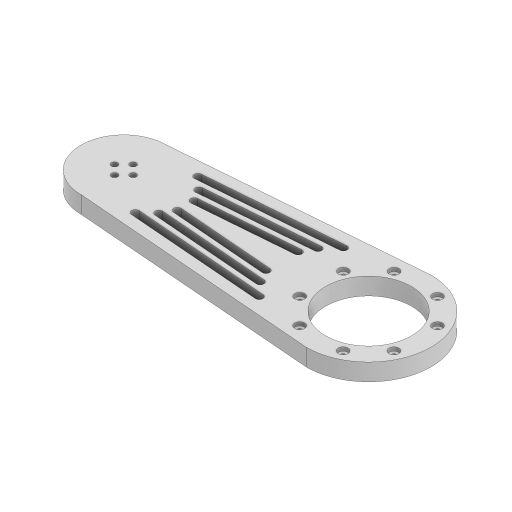
# Autodesk Inventor part: Link1
Saved by Autodesk Inventor 2024.3 (Build 283343000, 343)
## iProperties
Created: 2025-09-03
Part Number: Link1
Material: Generic
Document SubType Name: Modeling
Designer: danie
Density: 1 g/cm^3
Appearance: Default
Author: danie
Autodesk Inventor part; units mm, degrees
ref_plane "YZ Plane" through (0, 0, 0) normal (1, 0, 0) x (0, 1, 0)
ref_plane "XZ Plane" through (0, 0, 0) normal (0, 1, 0) x (-1, 0, 0)
ref_plane "XY Plane" through (0, 0, 0) normal (0, 0, 1) x (1, 0, 0)
sketch "Block1" plane through (0, 0, 0) normal (0, 0, 1) x (1, 0, 0)
  circle A0 centre (7.5478, 0.0598) radius 3.1
  circle A1 centre (-7.6522, 0.0598) radius 3.1
  circle A2 centre (-0.0522, 0.0598) radius 15.1
  circle A3 centre (-0.0522, 7.6598) radius 3.1
  circle A4 centre (-0.0522, -7.5402) radius 3.1
  point P0 (-0.0522, 0.0598)
sketch "Block2" plane through (0, 0, 0) normal (0, 0, 1) x (1, 0, 0)
  arc A0 (-125.615, -182.0442) -> (-128.3642, -184.6132) centre (-121.6807, -189.0099) ccw
  circle A1 centre (-125.7842, -178.7986) radius 1.5875
  circle A2 centre (-125.7842, -178.7986) radius 1.5875
  arc A3 (-123.2766, -176.7312) -> (-125.615, -182.0442) centre (-125.7842, -178.7986) ccw
  circle A4 centre (-125.7842, -178.7986) radius 3.25
  arc A5 (-140.9961, -137.689) -> (-141.0844, -134.7775) centre (-142.4103, -136.2748) ccw
  arc A6 (-128.2959, -137.4522) -> (-140.6552, -125.0571) centre (-164.2878, -160.9806) ccw
  arc A7 (-141.0844, -134.7775) -> (-153.1968, -127.7844) centre (-164.2878, -160.9806) ccw
  arc A8 (-143.2242, -122.3079) -> (-140.6552, -125.0571) centre (-136.2585, -118.3736) ccw
  circle A9 centre (-146.4698, -122.4771) radius 1.5875
  circle A10 centre (-146.4698, -122.4771) radius 1.5875
  arc A11 (-148.4415, -119.8935) -> (-143.2242, -122.3079) centre (-146.4698, -122.4771) ccw
  circle A12 centre (-146.4698, -122.4771) radius 3.25
  arc A13 (-152.1999, -119.7146) -> (-148.4415, -119.8935) centre (-149.951, -112.0372) ccw
  arc A14 (-202.9605, -139.9171) -> (-200.2113, -137.3481) centre (-206.8948, -132.9514) ccw
  circle A15 centre (-202.7913, -143.1627) radius 1.5875
  circle A16 centre (-202.7913, -143.1627) radius 1.5875
  arc A17 (-205.3749, -145.1344) -> (-202.9605, -139.9171) centre (-202.7913, -143.1627) ccw
  circle A18 centre (-202.7913, -143.1627) radius 3.25
  arc A19 (-150.7156, -144.8249) -> (-148.0149, -144.7078) centre (-149.4291, -143.2936) ccw
  line L0 (-140.9961, -137.689) -> (-148.0149, -144.7078)
  line L1 (-142.0587, -155.0244) -> (-132.4708, -152.4553)
  arc A20 (-142.0587, -155.0244) -> (-143.5104, -157.3047) centre (-141.541, -156.9562) ccw
  arc A21 (-177.8599, -177.1363) -> (-180.5606, -177.2535) centre (-179.1464, -178.6677) ccw
  arc A22 (-176.3756, -202.2467) -> (-180.134, -202.0677) centre (-178.6245, -209.924) ccw
  arc A23 (-175.3787, -194.1769) -> (-172.8131, -192.7976) centre (-174.7449, -192.28) ccw
  arc A24 (-177.8599, -177.1363) -> (-171.4929, -180.8123) centre (-164.2878, -160.9806) ccw
  line L2 (-170.244, -183.2097) -> (-172.8131, -192.7976)
  arc A25 (-170.244, -183.2097) -> (-171.4929, -180.8123) centre (-172.1759, -182.6921) ccw
  arc A26 (-157.0826, -180.8123) -> (-158.3315, -183.2097) centre (-156.3996, -182.6921) ccw
  line L3 (-155.7624, -192.7976) -> (-158.3315, -183.2097)
  arc A27 (-157.0826, -180.8123) -> (-150.7156, -177.1363) centre (-164.2878, -160.9806) ccw
  arc A28 (-155.7624, -192.7976) -> (-153.1968, -194.1769) centre (-153.8306, -192.28) ccw
  arc A29 (-176.3756, -202.2467) -> (-152.3193, -202.2815) centre (-164.2878, -160.9806) ccw
  arc A30 (-200.2796, -184.5091) -> (-203.4208, -181.7197) centre (-206.9757, -188.8865) ccw
  circle A31 centre (-202.8427, -178.6871) radius 1.5875
  arc A32 (-205.5197, -177.1495) -> (-205.5886, -172.9491) centre (-213.2724, -175.1758) ccw
  arc A33 (-205.5197, -177.1495) -> (-203.4208, -181.7197) centre (-201.6434, -178.1363) ccw
  arc A34 (-187.712, -124.9209) -> (-200.2113, -137.3481) centre (-164.2878, -160.9806) ccw
  arc A35 (-187.4911, -134.7775) -> (-187.5794, -137.689) centre (-186.1652, -136.2748) ccw
  line L4 (-180.5606, -144.7078) -> (-187.5794, -137.689)
  arc A36 (-180.5606, -144.7078) -> (-177.8599, -144.8249) centre (-179.1464, -143.2936) ccw
  arc A37 (-171.4929, -141.149) -> (-177.8599, -144.8249) centre (-164.2878, -160.9806) ccw
  arc A38 (-175.3787, -127.7844) -> (-187.4911, -134.7775) centre (-164.2878, -160.9806) ccw
  arc A39 (-171.4929, -141.149) -> (-170.244, -138.7515) centre (-172.1759, -139.2692) ccw
  arc A40 (-172.8131, -129.1637) -> (-175.3787, -127.7844) centre (-174.7449, -129.6813) ccw
  line L5 (-172.8131, -129.1637) -> (-170.244, -138.7515)
  arc A41 (-140.8512, -197.0324) -> (-128.3642, -184.6132) centre (-164.2878, -160.9806) ccw
  arc A42 (-141.0844, -187.1838) -> (-140.9961, -184.2723) centre (-142.4103, -185.6865) ccw
  line L6 (-148.0149, -177.2535) -> (-140.9961, -184.2723)
  arc A43 (-148.0149, -177.2535) -> (-150.7156, -177.1363) centre (-149.4291, -178.6677) ccw
  arc A44 (-140.8512, -197.0324) -> (-143.6285, -200.1265) centre (-136.4909, -203.7397) ccw
  arc A45 (-153.1968, -194.1769) -> (-141.0844, -187.1838) centre (-164.2878, -160.9806) ccw
  circle A46 centre (-146.5813, -199.5355) radius 1.5875
  arc A47 (-148.1624, -202.2017) -> (-143.6285, -200.1265) centre (-147.1972, -198.3199) ccw
  arc A48 (-148.1624, -202.2017) -> (-152.3193, -202.2815) centre (-150.0927, -209.9653) ccw
  arc A49 (-150.7156, -144.8249) -> (-157.0826, -141.149) centre (-164.2878, -160.9806) ccw
  arc A50 (-158.3315, -138.7515) -> (-157.0826, -141.149) centre (-156.3996, -139.2692) ccw
  line L7 (-158.3315, -138.7515) -> (-155.7624, -129.1637)
  arc A51 (-153.1968, -127.7844) -> (-155.7624, -129.1637) centre (-153.8306, -129.6813) ccw
  arc A52 (-187.712, -124.9209) -> (-184.9593, -121.878) centre (-192.07, -118.2121) ccw
  circle A53 centre (-181.9942, -122.4257) radius 1.5875
  arc A54 (-180.4775, -119.8197) -> (-184.9593, -121.878) centre (-181.404, -123.7109) ccw
  arc A55 (-180.4775, -119.8197) -> (-176.3756, -119.7146) centre (-178.6245, -112.0372) ccw
  arc A56 (-152.1999, -119.7146) -> (-176.3756, -119.7146) centre (-164.2878, -160.9806) ccw
  arc A57 (-128.2959, -137.4522) -> (-125.1547, -140.2416) centre (-121.5998, -133.0748) ccw
  circle A58 centre (-125.7329, -143.2742) radius 1.5875
  arc A59 (-123.0558, -144.8118) -> (-125.1547, -140.2416) centre (-126.9321, -143.8249) ccw
  arc A60 (-123.0558, -144.8118) -> (-122.9869, -149.0122) centre (-115.3031, -146.7855) ccw
  line L8 (-132.4708, -169.506) -> (-142.0587, -166.9369)
  arc A61 (-143.5104, -164.6566) -> (-142.0587, -166.9369) centre (-141.541, -165.0051) ccw
  arc A62 (-143.5104, -164.6566) -> (-143.5104, -157.3047) centre (-164.2878, -160.9806) ccw
  arc A63 (-129.9935, -153.9876) -> (-132.4708, -152.4553) centre (-131.9532, -154.3872) ccw
  arc A64 (-129.9935, -167.9737) -> (-129.9935, -153.9876) centre (-164.2878, -160.9806) ccw
  arc A65 (-132.4708, -169.506) -> (-129.9935, -167.9737) centre (-131.9532, -167.5741) ccw
  arc A66 (-123.0527, -173.1738) -> (-122.9869, -149.0122) centre (-164.2878, -160.9806) ccw
  arc A67 (-123.0527, -173.1738) -> (-123.2766, -176.7312) centre (-115.3811, -175.4423) ccw
  arc A68 (-205.5538, -148.8928) -> (-205.3749, -145.1344) centre (-213.2312, -146.6439) ccw
  arc A69 (-196.1047, -152.4553) -> (-198.582, -153.9876) centre (-196.6224, -154.3872) ccw
  line L9 (-196.1047, -152.4553) -> (-186.5169, -155.0244)
  arc A70 (-185.0651, -157.3047) -> (-186.5169, -155.0244) centre (-187.0345, -156.9562) ccw
  circle A71 centre (-164.2878, -160.9806) radius 15.5
  arc A72 (-185.0651, -157.3047) -> (-185.0651, -164.6566) centre (-164.2878, -160.9806) ccw
  arc A73 (-186.5169, -166.9369) -> (-185.0651, -164.6566) centre (-187.0345, -165.0051) ccw
  line L10 (-186.5169, -166.9369) -> (-196.1047, -169.506)
  arc A74 (-198.582, -153.9876) -> (-198.582, -167.9737) centre (-164.2878, -160.9806) ccw
  arc A75 (-205.5538, -148.8928) -> (-205.5886, -172.9491) centre (-164.2878, -160.9806) ccw
  arc A76 (-198.582, -167.9737) -> (-196.1047, -169.506) centre (-196.6224, -167.5741) ccw
  circle A77 centre (-182.1057, -199.4842) radius 1.5875
  circle A78 centre (-182.1057, -199.4842) radius 1.5875
  arc A79 (-187.4911, -187.1838) -> (-175.3787, -194.1769) centre (-164.2878, -160.9806) ccw
  arc A80 (-180.134, -202.0677) -> (-185.3513, -199.6534) centre (-182.1057, -199.4842) ccw
  circle A81 centre (-182.1057, -199.4842) radius 3.25
  arc A82 (-185.3513, -199.6534) -> (-187.9203, -196.9042) centre (-192.317, -203.5877) ccw
  arc A83 (-187.5794, -184.2723) -> (-187.4911, -187.1838) centre (-186.1652, -185.6865) ccw
  arc A84 (-200.2796, -184.5091) -> (-187.9203, -196.9042) centre (-164.2878, -160.9806) ccw
  line L11 (-187.5794, -184.2723) -> (-180.5606, -177.2535)
  point P0 (-164.2909, -160.9825)
sketch "Sketch1" plane through (0, 0, 0) normal (0, 1, 0) x (-1, 0, 0)
  circle A0 centre (0, 0) radius 15.1
  circle A1 centre (0, 0) radius 35
  line L0 (0, 0) -> (-200, 0)
  circle A2 centre (-200, 0) radius 15.5
  circle A3 centre (-200, 0) radius 51
  line L1 (0, 0) -> (0, 35)
  line L2 (0, 0) -> (0, -35)
  line L3 (-200, 0) -> (-200, 51)
  line L4 (-200, 0) -> (-200, -51)
  line L5 (0, 35) -> (-200, 51)
  line L6 (0, -35) -> (-200, -51)
  line L7 (-35, 25.6) -> (-145, 34.4) construction
  line L8 (-35.2392, 22.6096) -> (-145.2392, 31.4096)
  line L9 (-144.7608, 37.3904) -> (-34.7608, 28.5904)
  arc A4 (-35.2392, 22.6096) -> (-34.7608, 28.5904) centre (-35, 25.6) ccw
  arc A5 (-144.7608, 37.3904) -> (-145.2392, 31.4096) centre (-145, 34.4) ccw
  line L10 (-45, 16.4) -> (-135, 23.6) construction
  line L11 (-44.7608, 19.3904) -> (-134.7608, 26.5904)
  line L12 (-135.2392, 20.6096) -> (-45.2392, 13.4096)
  arc A6 (-45.2392, 13.4096) -> (-44.7608, 19.3904) centre (-45, 16.4) ccw
  arc A7 (-134.7608, 26.5904) -> (-135.2392, 20.6096) centre (-135, 23.6) ccw
  line L13 (-50.6641, 6.8531) -> (-129.3359, 13.1469) construction
  line L14 (-50.4249, 9.8436) -> (-129.0966, 16.1373)
  line L15 (-129.5751, 10.1564) -> (-50.9034, 3.8627)
  arc A8 (-50.9034, 3.8627) -> (-50.4249, 9.8436) centre (-50.6641, 6.8531) ccw
  arc A9 (-129.0966, 16.1373) -> (-129.5751, 10.1564) centre (-129.3359, 13.1469) ccw
  line L16 (-35.2392, -22.6096) -> (-145.2392, -31.4096)
  line L17 (-144.7608, -37.3904) -> (-34.7608, -28.5904)
  arc A10 (-34.7608, -28.5904) -> (-35.2392, -22.6096) centre (-35, -25.6) ccw
  arc A11 (-145.2392, -31.4096) -> (-144.7608, -37.3904) centre (-145, -34.4) ccw
  line L18 (-44.7608, -19.3904) -> (-134.7608, -26.5904)
  line L19 (-135.2392, -20.6096) -> (-45.2392, -13.4096)
  arc A12 (-44.7608, -19.3904) -> (-45.2392, -13.4096) centre (-45, -16.4) ccw
  arc A13 (-135.2392, -20.6096) -> (-134.7608, -26.5904) centre (-135, -23.6) ccw
  line L20 (-50.4249, -9.8436) -> (-129.0966, -16.1373)
  line L21 (-129.5751, -10.1564) -> (-50.9034, -3.8627)
  arc A14 (-50.4249, -9.8436) -> (-50.9034, -3.8627) centre (-50.6641, -6.8531) ccw
  arc A15 (-129.5751, -10.1564) -> (-129.0966, -16.1373) centre (-129.3359, -13.1469) ccw
  circle A16 centre (-200, 0) radius 35
  circle A17 centre (7.6, 0) radius 1.5
  circle A18 centre (0, 7.6) radius 1.5
  circle A19 centre (-7.6, 0) radius 1.5
  circle A20 centre (0, -7.6) radius 1.5
  circle A21 centre (7.6, 0) radius 3.1
  circle A22 centre (-7.6, 0) radius 3.1
  circle A23 centre (0, 0) radius 15.1
  circle A24 centre (0, 7.6) radius 3.1
  circle A25 centre (0, -7.6) radius 3.1
  arc A26 (-161.3273, -21.0635) -> (-164.0764, -23.6325) centre (-157.393, -28.0293) ccw
  circle A27 centre (-161.4965, -17.8179) radius 1.5875
  circle A28 centre (-161.4965, -17.8179) radius 1.5875
  arc A29 (-158.9888, -15.7505) -> (-161.3273, -21.0635) centre (-161.4965, -17.8179) ccw
  circle A30 centre (-161.4965, -17.8179) radius 3.25
  arc A31 (-176.7084, 23.2916) -> (-176.7967, 26.2032) centre (-178.1226, 24.7058) ccw
  arc A32 (-164.0082, 23.5285) -> (-176.3675, 35.9236) centre (-200, 0) ccw
  arc A33 (-176.7967, 26.2032) -> (-188.9091, 33.1962) centre (-200, 0) ccw
  arc A34 (-178.9365, 38.6727) -> (-176.3675, 35.9236) centre (-171.9707, 42.607) ccw
  circle A35 centre (-182.1821, 38.5035) radius 1.5875
  circle A36 centre (-182.1821, 38.5035) radius 1.5875
  arc A37 (-184.1537, 41.0871) -> (-178.9365, 38.6727) centre (-182.1821, 38.5035) ccw
  circle A38 centre (-182.1821, 38.5035) radius 3.25
  arc A39 (-187.9121, 41.266) -> (-184.1537, 41.0871) centre (-185.6632, 48.9434) ccw
  arc A40 (-238.6727, 21.0635) -> (-235.9236, 23.6325) centre (-242.607, 28.0293) ccw
  circle A41 centre (-238.5035, 17.8179) radius 1.5875
  circle A42 centre (-238.5035, 17.8179) radius 1.5875
  arc A43 (-241.0871, 15.8463) -> (-238.6727, 21.0635) centre (-238.5035, 17.8179) ccw
  circle A44 centre (-238.5035, 17.8179) radius 3.25
  arc A45 (-186.4278, 16.1557) -> (-183.7272, 16.2728) centre (-185.1414, 17.687) ccw
  line L22 (-176.7084, 23.2916) -> (-183.7272, 16.2728)
  line L23 (-177.7709, 5.9563) -> (-168.183, 8.5253)
  arc A46 (-177.7709, 5.9563) -> (-179.2227, 3.676) centre (-177.2533, 4.0244) ccw
  arc A47 (-213.5722, -16.1557) -> (-216.2728, -16.2728) centre (-214.8586, -17.687) ccw
  arc A48 (-212.0879, -41.266) -> (-215.8463, -41.0871) centre (-214.3368, -48.9434) ccw
  arc A49 (-211.0909, -33.1962) -> (-208.5253, -31.817) centre (-210.4572, -31.2993) ccw
  arc A50 (-213.5722, -16.1557) -> (-207.2052, -19.8317) centre (-200, 0) ccw
  line L24 (-205.9563, -22.2291) -> (-208.5253, -31.817)
  arc A51 (-205.9563, -22.2291) -> (-207.2052, -19.8317) centre (-207.8881, -21.7115) ccw
  arc A52 (-192.7948, -19.8317) -> (-194.0437, -22.2291) centre (-192.1119, -21.7115) ccw
  line L25 (-191.4747, -31.817) -> (-194.0437, -22.2291)
  arc A53 (-192.7948, -19.8317) -> (-186.4278, -16.1557) centre (-200, 0) ccw
  arc A54 (-191.4747, -31.817) -> (-188.9091, -33.1962) centre (-189.5428, -31.2993) ccw
  arc A55 (-212.0879, -41.266) -> (-188.0316, -41.3008) centre (-200, 0) ccw
  arc A56 (-235.9918, -23.5285) -> (-239.1331, -20.7391) centre (-242.688, -27.9059) ccw
  circle A57 centre (-238.5549, -17.7065) radius 1.5875
  arc A58 (-241.232, -16.1688) -> (-241.3008, -11.9684) centre (-248.9847, -14.1951) ccw
  arc A59 (-241.232, -16.1688) -> (-239.1331, -20.7391) centre (-237.3556, -17.1557) ccw
  arc A60 (-223.4243, 36.0597) -> (-235.9236, 23.6325) centre (-200, 0) ccw
  arc A61 (-223.2033, 26.2032) -> (-223.2916, 23.2916) centre (-221.8774, 24.7058) ccw
  line L26 (-216.2728, 16.2728) -> (-223.2916, 23.2916)
  arc A62 (-216.2728, 16.2728) -> (-213.5722, 16.1557) centre (-214.8586, 17.687) ccw
  arc A63 (-207.2052, 19.8317) -> (-213.5722, 16.1557) centre (-200, 0) ccw
  arc A64 (-211.0909, 33.1962) -> (-223.2033, 26.2032) centre (-200, 0) ccw
  arc A65 (-207.2052, 19.8317) -> (-205.9563, 22.2291) centre (-207.8881, 21.7115) ccw
  arc A66 (-208.5253, 31.817) -> (-211.0909, 33.1962) centre (-210.4572, 31.2993) ccw
  line L27 (-208.5253, 31.817) -> (-205.9563, 22.2291)
  arc A67 (-176.5634, -36.0517) -> (-164.0764, -23.6325) centre (-200, 0) ccw
  arc A68 (-176.7967, -26.2032) -> (-176.7084, -23.2916) centre (-178.1226, -24.7058) ccw
  line L28 (-183.7272, -16.2728) -> (-176.7084, -23.2916)
  arc A69 (-183.7272, -16.2728) -> (-186.4278, -16.1557) centre (-185.1414, -17.687) ccw
  arc A70 (-176.5634, -36.0517) -> (-179.3407, -39.1458) centre (-172.2032, -42.759) ccw
  arc A71 (-188.9091, -33.1962) -> (-176.7967, -26.2032) centre (-200, 0) ccw
  circle A72 centre (-182.2935, -38.5549) radius 1.5875
  arc A73 (-183.8746, -41.221) -> (-179.3407, -39.1458) centre (-182.9095, -37.3392) ccw
  arc A74 (-183.8746, -41.221) -> (-188.0316, -41.3008) centre (-185.8049, -48.9847) ccw
  arc A75 (-186.4278, 16.1557) -> (-192.7948, 19.8317) centre (-200, 0) ccw
  arc A76 (-194.0437, 22.2291) -> (-192.7948, 19.8317) centre (-192.1119, 21.7115) ccw
  line L29 (-194.0437, 22.2291) -> (-191.4747, 31.817)
  arc A77 (-188.9091, 33.1962) -> (-191.4747, 31.817) centre (-189.5428, 31.2993) ccw
  arc A78 (-223.4243, 36.0597) -> (-220.6716, 39.1027) centre (-227.7823, 42.7685) ccw
  circle A79 centre (-217.7065, 38.5549) radius 1.5875
  arc A80 (-216.1898, 41.161) -> (-220.6716, 39.1027) centre (-217.1163, 37.2697) ccw
  arc A81 (-216.1898, 41.161) -> (-212.0879, 41.266) centre (-214.3368, 48.9434) ccw
  arc A82 (-187.9121, 41.266) -> (-212.0879, 41.266) centre (-200, 0) ccw
  arc A83 (-164.0082, 23.5285) -> (-160.8669, 20.7391) centre (-157.312, 27.9059) ccw
  circle A84 centre (-161.4451, 17.7065) radius 1.5875
  arc A85 (-158.768, 16.1688) -> (-160.8669, 20.7391) centre (-162.6444, 17.1557) ccw
  arc A86 (-158.768, 16.1688) -> (-158.6992, 11.9684) centre (-151.0153, 14.1951) ccw
  line L30 (-168.183, -8.5253) -> (-177.7709, -5.9563)
  arc A87 (-179.2227, -3.676) -> (-177.7709, -5.9563) centre (-177.2533, -4.0244) ccw
  arc A88 (-179.2227, -3.676) -> (-179.2227, 3.676) centre (-200, 0) ccw
  arc A89 (-165.7057, 6.9931) -> (-168.183, 8.5253) centre (-167.6654, 6.5935) ccw
  arc A90 (-165.7057, -6.9931) -> (-165.7057, 6.9931) centre (-200, 0) ccw
  arc A91 (-168.183, -8.5253) -> (-165.7057, -6.9931) centre (-167.6654, -6.5935) ccw
  arc A92 (-158.765, -12.1931) -> (-158.6992, 11.9684) centre (-200, 0) ccw
  arc A93 (-158.765, -12.1931) -> (-158.9888, -15.7505) centre (-151.0933, -14.4616) ccw
  arc A94 (-241.266, 12.0879) -> (-241.0871, 15.8463) centre (-248.9434, 14.3368) ccw
  arc A95 (-231.817, 8.5253) -> (-234.2943, 6.9931) centre (-232.3346, 6.5935) ccw
  line L31 (-231.817, 8.5253) -> (-222.2291, 5.9563)
  arc A96 (-220.7773, 3.676) -> (-222.2291, 5.9563) centre (-222.7467, 4.0244) ccw
  circle A97 centre (-200, 0) radius 15.5
  arc A98 (-220.7773, 3.676) -> (-220.7773, -3.676) centre (-200, 0) ccw
  arc A99 (-222.2291, -5.9563) -> (-220.7773, -3.676) centre (-222.7467, -4.0244) ccw
  line L32 (-222.2291, -5.9563) -> (-231.817, -8.5253)
  arc A100 (-234.2943, 6.9931) -> (-234.2943, -6.9931) centre (-200, 0) ccw
  arc A101 (-241.266, 12.0879) -> (-241.3008, -11.9684) centre (-200, 0) ccw
  arc A102 (-234.2943, -6.9931) -> (-231.817, -8.5253) centre (-232.3346, -6.5935) ccw
  circle A103 centre (-217.8179, -38.5035) radius 1.5875
  circle A104 centre (-217.8179, -38.5035) radius 1.5875
  arc A105 (-223.2033, -26.2032) -> (-211.0909, -33.1962) centre (-200, 0) ccw
  arc A106 (-215.8463, -41.0871) -> (-221.0635, -38.6727) centre (-217.8179, -38.5035) ccw
  circle A107 centre (-217.8179, -38.5035) radius 3.25
  arc A108 (-221.0635, -38.6727) -> (-223.6325, -35.9236) centre (-228.0293, -42.607) ccw
  arc A109 (-223.2916, -23.2916) -> (-223.2033, -26.2032) centre (-221.8774, -24.7058) ccw
  arc A110 (-235.9918, -23.5285) -> (-223.6325, -35.9236) centre (-200, 0) ccw
  line L33 (-223.2916, -23.2916) -> (-216.2728, -16.2728)
  point P0 (-90, 30)
  point P1 (-90, 20)
  point P2 (-90, 10)
  point P3 (-161.3273, -21.0635)
  point P4 (-158.9888, -15.7505)
  point P5 (-215.8463, -41.0871)
  point P6 (-221.0635, -38.6727)
  point P7 (-241.0871, 15.8463)
  point P8 (-178.9365, 38.6727)
  point P9 (-184.1537, 41.0871)
  point P10 (-211.0909, -33.1962)
  point P11 (-223.2033, -26.2032)
  point P12 (-234.2943, -6.9931)
  point P13 (-234.2943, 6.9931)
  point P14 (-223.2033, 26.2032)
  point P15 (-211.0909, 33.1962)
  point P16 (-188.9091, 33.1962)
  point P17 (-176.7967, 26.2032)
  point P18 (-165.7057, 6.9931)
  point P19 (-165.7057, -6.9931)
  point P20 (-176.7967, -26.2032)
  point P21 (-188.9091, -33.1962)
  dimension "d0" = 70
  dimension "d1" = 200
  dimension "d2" = 30
  dimension "d3" = 6
  dimension "d4" = 110
  dimension "d5" = 6
  dimension "d6" = 90
  dimension "d7" = 90
  dimension "d8" = 90
  dimension "d9" = 90
  dimension "d10" = 6
  dimension "d11" = 10
  dimension "d12" = 10
  dimension "d15" = 3
  dimension "d16" = 3
  dimension "d17" = 3
  dimension "d18" = 3
  constraints: 50 end point, 28 point on circle, 21 centre point, 18 symmetric about line, 12 tangent, 6 parallel, 3 coincident, 3 midpoint, 3 vertical, 1 horizontal, 1 point on line, 17 other
  measures "d0" diameter of A1
  measures "d1" distance of L0.start L0.end
  measures "d2" distance from line of L0 point (-90, 30)
  measures "d3" distance between parallel lines of L8 L9
  measures "d4" horizontal distance of L7.end L7.start
  measures "d5" distance between parallel lines of L12 L11
  measures "d6" horizontal distance of L10.end L10.start
  measures "d10" distance between parallel lines of L15 L14
  measures "d11" distance of point (-90, 30) point (-90, 20)
  measures "d12" distance of point (-90, 10) point (-90, 20)
  measures "d15" diameter of A17
  measures "d16" diameter of A18
  measures "d17" diameter of A19
  measures "d18" diameter of A20
extrude "Extrusion1" add sketch "Sketch1" along normal blind 14 contours A0 L2 A25 L1 A24 | A0 L1 A1 L2 | L1 A24 L0 A22 A0 | A0 L0 A1 L1 | L2 A1 L0 A0 | A0 L0 A22 L2 A25 | A24 L1 A18 | L1 A18 A24 | A1 L0 A3 L5 | A25 L2 A20 | L2 A20 A25 | L6 A3 L0 A1 | A22 L0 A19 | L0 A19 A22 | A3 L0 A92 A86 A85 A83 A32 A34 A38 A39 A82 L3 L5 | L6 L4 A55 A74 A73 A70 A67 A26 A30 A93 A92 L0 A3 | L3 A82 A81 A80 A78 A60 A40 A44 A94 A101 A58 A59 A56 A110 A108 A107 A48 A55 L4 A3 | A92 A93 A29 A26 A67 A70 A73 A74 A55 L4 A16 L0 | L0 A16 L3 A82 A39 A37 A34 A32 A83 A85 A86 A92 | L3 A16 L4 A55 A48 A106 A108 A110 A56 A59 A58 A101 A94 A43 A40 A60 A78 A80 A81 A82 | A30 A29 | A38 A37 | A107 A106 | A43 A44 | A21
sketch "Sketch2" plane through (0, 14, 0) normal (0, 1, 0) x (1, 0, 0)
  circle A0 centre (217.8179, 38.5035) radius 1.5875 projected
  circle A1 centre (161.4965, 17.8179) radius 1.5875 projected
  arc A2 (200, -51) -> (200, 51) centre (200, 0) ccw projected
  line L0 (200, 51) -> (0, 35) projected
  arc A3 (0, 35) -> (0, -35) centre (0, 0) ccw projected
  line L1 (0, -35) -> (200, -51) projected
  circle A4 centre (0, -7.6) radius 1.5 projected
  circle A5 centre (-7.6, 0) radius 1.5 projected
  circle A6 centre (161.4451, -17.7065) radius 1.5875 projected
  circle A7 centre (217.7065, -38.5549) radius 1.5875 projected
  circle A8 centre (238.5549, 17.7065) radius 1.5875 projected
  circle A9 centre (182.2935, 38.5549) radius 1.5875 projected
  circle A10 centre (200, 0) radius 35 projected
  line L2 (129.5751, 10.1564) -> (50.9034, 3.8627) projected
  arc A11 (50.4249, 9.8436) -> (50.9034, 3.8627) centre (50.6641, 6.8531) ccw projected
  line L3 (50.4249, 9.8436) -> (129.0966, 16.1373) projected
  arc A12 (129.5751, 10.1564) -> (129.0966, 16.1373) centre (129.3359, 13.1469) ccw projected
  line L4 (44.7608, 19.3904) -> (134.7608, 26.5904) projected
  arc A13 (135.2392, 20.6096) -> (134.7608, 26.5904) centre (135, 23.6) ccw projected
  line L5 (135.2392, 20.6096) -> (45.2392, 13.4096) projected
  arc A14 (44.7608, 19.3904) -> (45.2392, 13.4096) centre (45, 16.4) ccw projected
  arc A15 (34.7608, 28.5904) -> (35.2392, 22.6096) centre (35, 25.6) ccw projected
  line L6 (34.7608, 28.5904) -> (144.7608, 37.3904) projected
  arc A16 (145.2392, 31.4096) -> (144.7608, 37.3904) centre (145, 34.4) ccw projected
  line L7 (145.2392, 31.4096) -> (35.2392, 22.6096) projected
  line L8 (144.7608, -37.3904) -> (34.7608, -28.5904) projected
  arc A17 (35.2392, -22.6096) -> (34.7608, -28.5904) centre (35, -25.6) ccw projected
  line L9 (35.2392, -22.6096) -> (145.2392, -31.4096) projected
  arc A18 (144.7608, -37.3904) -> (145.2392, -31.4096) centre (145, -34.4) ccw projected
  arc A19 (45.2392, -13.4096) -> (44.7608, -19.3904) centre (45, -16.4) ccw projected
  line L10 (45.2392, -13.4096) -> (135.2392, -20.6096) projected
  arc A20 (134.7608, -26.5904) -> (135.2392, -20.6096) centre (135, -23.6) ccw projected
  line L11 (134.7608, -26.5904) -> (44.7608, -19.3904) projected
  arc A21 (50.9034, -3.8627) -> (50.4249, -9.8436) centre (50.6641, -6.8531) ccw projected
  line L12 (50.9034, -3.8627) -> (129.5751, -10.1564) projected
  arc A22 (129.0966, -16.1373) -> (129.5751, -10.1564) centre (129.3359, -13.1469) ccw projected
  line L13 (129.0966, -16.1373) -> (50.4249, -9.8436) projected
  circle A23 centre (7.6, 0) radius 1.5 projected
  circle A24 centre (0, 7.6) radius 1.5 projected
  circle A25 centre (238.5035, -17.8179) radius 1.5875 projected
  circle A26 centre (182.1821, -38.5035) radius 1.5875 projected
hole "Hole1" at (161.4451, 14, 17.7065) at (182.1821, 14, 38.5035) at (217.7065, 14, 38.5549) at (238.5035, 14, 17.8179) at (238.5549, 14, -17.7065) at (217.8179, 14, -38.5035) at (182.2935, 14, -38.5549) at (161.4965, 14, -17.8179) direction (0, -1, 0) diameter 3.175 depth 50 tip angle 118 counterbore diameter 8 counterbore depth 3
hole "Hole2" at (0, 14, 7.6) at (-7.6, 14, 0) at (7.6, 14, 0) at (0, 14, -7.6) direction (0, -1, 0) diameter 3 depth 50 tip angle 118 counterbore diameter 5 counterbore depth 3
body "Solid1"
